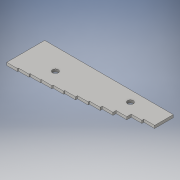
# Autodesk Inventor part: twinkle_twinkle_base
Saved by Autodesk Inventor 2016 (Build 200138000, 138)
## iProperties
Created: 2015-05-04
Part Number: twinkle_twinkle_base
Material: Generic
Document SubType Name: Modeling
Designer: Trevor
Density: 1 g/cm^3
Appearance: Default
Author: Trevor
## iProperties of the stored document twinkle_twinkle_base_3DPrint.ipt
Created: 2015-05-04
Part Number: twinkle_twinkle_base_3DPrint
Material: Generic
Document SubType Name: Modeling
Designer: Trevor
Density: 1 g/cm^3
Appearance: Default
Author: Trevor
Autodesk Inventor part; units mm, degrees
ref_plane "YZ Plane" through (0, 0, 0) normal (1, 0, 0) x (0, 1, 0)
ref_plane "XZ Plane" through (0, 0, 0) normal (0, 1, 0) x (-1, 0, 0)
ref_plane "XY Plane" through (0, 0, 0) normal (0, 0, 1) x (1, 0, 0)
sketch "Sketch1" plane through (0, 0, 0) normal (0, 1, 0) x (-1, 0, 0)
  line L0 (6.35, 11.0627) -> (0, 11.0627)
  line L1 (0, 11.0627) -> (0, 0)
  line L2 (0, 0) -> (76.2, 0)
  line L3 (6.35, 11.0627) -> (6.35, 12.2238)
  line L4 (6.35, 12.2238) -> (12.7, 12.2238)
  line L5 (12.7, 12.2238) -> (12.7, 14.8493)
  line L6 (12.7, 14.8493) -> (19.05, 14.8493)
  line L7 (19.05, 14.8493) -> (19.05, 16.6932)
  line L8 (19.05, 16.6932) -> (25.4, 16.6932)
  line L9 (25.4, 16.6932) -> (25.4, 17.9429)
  line L10 (25.4, 17.9429) -> (31.75, 17.9429)
  line L11 (31.75, 17.9429) -> (31.75, 18.7178)
  line L12 (31.75, 18.7178) -> (38.1, 18.7178)
  line L13 (38.1, 18.7178) -> (38.1, 19.7994)
  line L14 (38.1, 19.7994) -> (44.45, 19.7994)
  line L15 (44.45, 19.7994) -> (44.45, 20.4702)
  line L16 (44.45, 20.4702) -> (50.8, 20.4702)
  line L17 (50.8, 20.4702) -> (50.8, 21.1032)
  line L18 (50.8, 21.1032) -> (57.15, 21.1032)
  line L19 (57.15, 21.1032) -> (57.15, 21.4063)
  line L20 (57.15, 21.4063) -> (63.5, 21.4063)
  line L21 (63.5, 21.4063) -> (63.5, 21.9869)
  line L22 (63.5, 21.9869) -> (69.85, 21.9869)
  line L23 (69.85, 21.9869) -> (69.85, 22.5348)
  line L24 (69.85, 22.5348) -> (76.2, 22.5348)
  line L25 (76.2, 0) -> (76.2, 22.5348)
  circle A0 centre (19.05, 6.35) radius 1.7
  circle A1 centre (57.15, 12.7) radius 1.7
  constraints: 52 end point, 13 perpendicular, 12 parallel, 2 centre point, 1 equal radius
extrude "Extrusion1" add sketch "Sketch1" along normal blind 1.5875
body "Solid1"
